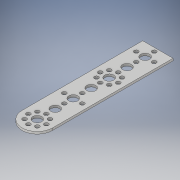
# Autodesk Inventor part: Tetrix Flat bar 160 mm
Saved by Autodesk Inventor 2019 (Build 230136000, 136)
## iProperties
Created: 2015-12-29
Part Number: Tetrix Flat bar 160 mm
Material: Generic
Document SubType Name: Modeling
Designer: Delta
Density: 1 g/cm^3
Appearance: Default
Author: Delta
Autodesk Inventor part; units mm, degrees
ref_plane "YZ Plane" through (0, 0, 0) normal (1, 0, 0) x (0, 1, 0)
ref_plane "XZ Plane" through (0, 0, 0) normal (0, 1, 0) x (-1, 0, 0)
ref_plane "XY Plane" through (0, 0, 0) normal (0, 0, 1) x (1, 0, 0)
sketch "Sketch1" plane through (0, 0, 0) normal (0, 1, 0) x (-1, 0, 0)
  arc A0 (-5.66, 120.49) -> (-5.66, 124.19) centre (-5.66, 122.34) ccw
  arc A1 (-5.66, 124.19) -> (-5.66, 120.49) centre (-5.66, 122.34) ccw
  arc A2 (5.66, 120.49) -> (5.66, 124.19) centre (5.66, 122.34) ccw
  arc A3 (5.66, 124.19) -> (5.66, 120.49) centre (5.66, 122.34) ccw
  arc A4 (0, 134.15) -> (0, 137.85) centre (0, 136) ccw
  arc A5 (0, 137.85) -> (0, 134.15) centre (0, 136) ccw
  arc A6 (-5.66, 131.81) -> (-5.66, 135.51) centre (-5.66, 133.66) ccw
  arc A7 (-5.66, 135.51) -> (-5.66, 131.81) centre (-5.66, 133.66) ccw
  arc A8 (5.66, 131.81) -> (5.66, 135.51) centre (5.66, 133.66) ccw
  arc A9 (5.66, 135.51) -> (5.66, 131.81) centre (5.66, 133.66) ccw
  arc A10 (8, 126.15) -> (8, 129.85) centre (8, 128) ccw
  arc A11 (8, 129.85) -> (8, 126.15) centre (8, 128) ccw
  arc A12 (0, 124) -> (0, 132) centre (0, 128) ccw
  arc A13 (0, 132) -> (0, 124) centre (0, 128) ccw
  arc A14 (-8, 126.15) -> (-8, 129.85) centre (-8, 128) ccw
  arc A15 (-8, 129.85) -> (-8, 126.15) centre (-8, 128) ccw
  arc A16 (0, 118.15) -> (0, 121.85) centre (0, 120) ccw
  arc A17 (0, 121.85) -> (0, 118.15) centre (0, 120) ccw
  arc A18 (-5.66, 195.81) -> (-5.66, 199.51) centre (-5.66, 197.66) ccw
  arc A19 (-5.66, 199.51) -> (-5.66, 195.81) centre (-5.66, 197.66) ccw
  arc A20 (-5.66, 184.49) -> (-5.66, 188.19) centre (-5.66, 186.34) ccw
  arc A21 (-5.66, 188.19) -> (-5.66, 184.49) centre (-5.66, 186.34) ccw
  arc A22 (5.66, 184.49) -> (5.66, 188.19) centre (5.66, 186.34) ccw
  arc A23 (5.66, 188.19) -> (5.66, 184.49) centre (5.66, 186.34) ccw
  arc A24 (5.66, 195.81) -> (5.66, 199.51) centre (5.66, 197.66) ccw
  arc A25 (5.66, 199.51) -> (5.66, 195.81) centre (5.66, 197.66) ccw
  arc A26 (8, 190.15) -> (8, 193.85) centre (8, 192) ccw
  arc A27 (8, 193.85) -> (8, 190.15) centre (8, 192) ccw
  arc A28 (-8, 190.15) -> (-8, 193.85) centre (-8, 192) ccw
  arc A29 (-8, 193.85) -> (-8, 190.15) centre (-8, 192) ccw
  arc A30 (0, 198.15) -> (0, 201.85) centre (0, 200) ccw
  arc A31 (0, 201.85) -> (0, 198.15) centre (0, 200) ccw
  arc A32 (0, 182.15) -> (0, 185.85) centre (0, 184) ccw
  arc A33 (0, 185.85) -> (0, 182.15) centre (0, 184) ccw
  arc A34 (0, 188) -> (0, 196) centre (0, 192) ccw
  arc A35 (0, 196) -> (0, 188) centre (0, 192) ccw
  arc A36 (8, 158.15) -> (8, 161.85) centre (8, 160) ccw
  arc A37 (8, 161.85) -> (8, 158.15) centre (8, 160) ccw
  arc A38 (-8, 158.15) -> (-8, 161.85) centre (-8, 160) ccw
  arc A39 (-8, 161.85) -> (-8, 158.15) centre (-8, 160) ccw
  arc A40 (0, 166.15) -> (0, 169.85) centre (0, 168) ccw
  arc A41 (0, 169.85) -> (0, 166.15) centre (0, 168) ccw
  arc A42 (0, 150.15) -> (0, 153.85) centre (0, 152) ccw
  arc A43 (0, 153.85) -> (0, 150.15) centre (0, 152) ccw
  arc A44 (0, 156) -> (0, 164) centre (0, 160) ccw
  arc A45 (0, 164) -> (0, 156) centre (0, 160) ccw
  arc A46 (-5.66, 248.49) -> (-5.66, 252.19) centre (-5.66, 250.34) ccw
  arc A47 (-5.66, 252.19) -> (-5.66, 248.49) centre (-5.66, 250.34) ccw
  arc A48 (5.66, 248.49) -> (5.66, 252.19) centre (5.66, 250.34) ccw
  arc A49 (5.66, 252.19) -> (5.66, 248.49) centre (5.66, 250.34) ccw
  arc A50 (0, 262.15) -> (0, 265.85) centre (0, 264) ccw
  arc A51 (0, 265.85) -> (0, 262.15) centre (0, 264) ccw
  arc A52 (-5.66, 259.81) -> (-5.66, 263.51) centre (-5.66, 261.66) ccw
  arc A53 (-5.66, 263.51) -> (-5.66, 259.81) centre (-5.66, 261.66) ccw
  arc A54 (5.66, 259.81) -> (5.66, 263.51) centre (5.66, 261.66) ccw
  arc A55 (5.66, 263.51) -> (5.66, 259.81) centre (5.66, 261.66) ccw
  arc A56 (8, 254.15) -> (8, 257.85) centre (8, 256) ccw
  arc A57 (8, 257.85) -> (8, 254.15) centre (8, 256) ccw
  arc A58 (0, 252) -> (0, 260) centre (0, 256) ccw
  arc A59 (0, 260) -> (0, 252) centre (0, 256) ccw
  arc A60 (8, 222.15) -> (8, 225.85) centre (8, 224) ccw
  arc A61 (8, 225.85) -> (8, 222.15) centre (8, 224) ccw
  arc A62 (-8, 222.15) -> (-8, 225.85) centre (-8, 224) ccw
  arc A63 (-8, 225.85) -> (-8, 222.15) centre (-8, 224) ccw
  arc A64 (0, 230.15) -> (0, 233.85) centre (0, 232) ccw
  arc A65 (0, 233.85) -> (0, 230.15) centre (0, 232) ccw
  arc A66 (0, 214.15) -> (0, 217.85) centre (0, 216) ccw
  arc A67 (0, 217.85) -> (0, 214.15) centre (0, 216) ccw
  arc A68 (0, 220) -> (0, 228) centre (0, 224) ccw
  arc A69 (0, 228) -> (0, 220) centre (0, 224) ccw
  arc A70 (0, 140) -> (0, 148) centre (0, 144) ccw
  arc A71 (0, 148) -> (0, 140) centre (0, 144) ccw
  arc A72 (0.1754, 172) -> (0.1754, 180) centre (0.1754, 176) ccw
  arc A73 (0.1754, 180) -> (0.1754, 172) centre (0.1754, 176) ccw
  arc A74 (0, 204) -> (0, 212) centre (0, 208) ccw
  arc A75 (0, 212) -> (0, 204) centre (0, 208) ccw
  arc A76 (0, 236) -> (0, 244) centre (0, 240) ccw
  arc A77 (0, 244) -> (0, 236) centre (0, 240) ccw
  arc A78 (-8, 254.15) -> (-8, 257.85) centre (-8, 256) ccw
  arc A79 (-8, 257.85) -> (-8, 254.15) centre (-8, 256) ccw
  arc A80 (0, 246.15) -> (0, 249.85) centre (0, 248) ccw
  arc A81 (0, 249.85) -> (0, 246.15) centre (0, 248) ccw
  arc A82 (13.5, 256) -> (0, 269.5) centre (0, 256) ccw
  arc A83 (0, 269.5) -> (-13.5, 256) centre (0, 256) ccw
  line L0 (-13.5, 256) -> (-13.5, 128)
  line L1 (13.5, 128) -> (13.5, 256)
  arc A84 (2.852, 141.1953) -> (-2.852, 141.1953) centre (0, 128) ccw
  arc A85 (-13.5, 128) -> (13.5, 128) centre (0, 128) ccw
  point P0 (0, 0)
  point P1 (0, 128)
  constraints: 174 point on circle, 86 centre point, 4 end point, 1 coincident
extrude "Extrusion1" add sketch "Sketch1" along normal blind 2
sketch "Sketch2" plane through (0, 2, 0) normal (0, 1, 0) x (1, 0, 0)
  line L0 (-13.5, -128) -> (-13.5, -256) projected
  line L1 (-13.5, -148.6948) -> (13.5, -148.6948)
  line L2 (13.5, -148.6948) -> (13.5, -110.804)
  line L3 (13.5, -110.804) -> (-13.5, -110.804)
  line L4 (-13.5, -110.804) -> (-13.5, -148.6948)
  point P0 (0, 0)
  constraints: 8 end point, 2 parallel, 1 horizontal, 1 perpendicular, 1 point on line
extrude "Extrusion2" cut sketch "Sketch2" against normal blind 25.4
body "Solid1"
